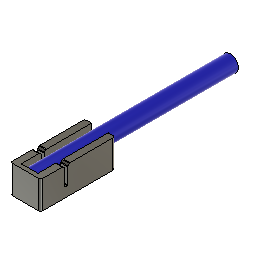
Prusa_MK3_Silicone-Leveling-Jig (Autodesk Fusion 360 design; units mm, degrees)
Autodesk Fusion 360 part; units mm, degrees
sketch "Sketch1" plane through (0, 0, 0) normal (0, 1, 0) x (1, 0, 0)
  circle A0 centre (0, 0) radius 4
  circle A1 centre (0, 0) radius 1.5
  dimension "d1" = 8
  dimension "d2" = 3
  constraint coincident A0.centre A1.centre
  measures "d1" diameter of A0
  measures "d2" diameter of A1
extrude "Extrude1" add sketch "Sketch1" along normal blind 100 makes body 1
sketch "Sketch2" plane through (0, 0, 0) normal (0, 1, 0) x (1, 0, 0)
  circle A0 centre (0, 0) radius 4.15
  line L0 (0, 0) -> (7.5, 0)
  line L1 (7.5, 0) -> (7.5, -7.5)
  line L2 (7.5, -7.5) -> (0, -7.5)
  line L3 (0, -7.5) -> (0, 0)
  line L4 (0, 0) -> (-7.5, 0)
  line L5 (-7.5, 0) -> (-7.5, 7.5)
  line L6 (-7.5, 7.5) -> (0, 7.5)
  line L7 (0, 7.5) -> (0, 0)
  line L8 (-7.5, 7.5) -> (7.5, 7.5)
  line L9 (7.5, 7.5) -> (7.5, -7.5)
  line L10 (7.5, -7.5) -> (-7.5, -7.5)
  line L11 (-7.5, -7.5) -> (-7.5, 7.5)
  dimension "d5" = 8.3
  dimension "d6" = 7.5
  dimension "d7" = 7.5
  dimension "d8" = 7.5
  constraint coincident A0.centre L0.start
  constraint horizontal L0
  constraint vertical L1
  constraint horizontal L2
  constraint vertical L3
  constraint horizontal L4
  constraint vertical L5
  constraint horizontal L6
  constraint vertical L7
  constraint horizontal L8
  constraint vertical L9
  constraint horizontal L10
  constraint vertical L11
  measures "d5" diameter of A0
  measures "d6" distance of A0.centre L0.end
  measures "d7" distance of A0.centre L4.end
  measures "d8" distance of A0.centre L6.end
extrude "Extrude2" add sketch "Sketch2" along normal blind 35 separate body contours A0 L0 L7 L8 L9 | A0 L4 L5 L6 L7 L8 L11 makes body 2
extrude "Extrude3" add 2 faces at (5.2667, 11.6667, 0) (-5.2667, 23.3333, 0) along direction (0, 0, 1) blind 4.5 on bodies 2 bodies 2
sketch "Sketch3" plane through (0, 0, 0) normal (0, -1, 0) x (1, 0, 0)
  arc A0 (-4.15, 0) -> (4.15, 0) centre (0, 0) ccw
  line L0 (-4.15, 0) -> (-4.15, 4.5)
  line L1 (-4.15, 4.5) -> (-7.5, 4.5)
  line L2 (-7.5, 4.5) -> (-7.5, -7.5)
  line L3 (-7.5, -7.5) -> (7.5, -7.5)
  line L4 (7.5, -7.5) -> (7.5, 4.5)
  line L5 (7.5, 4.5) -> (4.15, 4.5)
  line L6 (4.15, 4.5) -> (4.15, 0)
  line L7 (7.5, -7.5) -> (-7.5, -7.5)
  line L8 (-7.5, -7.5) -> (-7.5, 4.5)
  line L9 (-7.5, 4.5) -> (7.5, 4.5)
  line L10 (7.5, 4.5) -> (7.5, -7.5)
  constraint horizontal L7
  constraint vertical L8
  constraint horizontal L9
  constraint vertical L10
  constraint coincident L1.end L2.start
  constraint coincident L3.end L4.start
extrude "Extrude4" add sketch "Sketch3" along normal blind 2 bodies 2
sketch "Sketch4" plane through (0, 0, 4.5) normal (0, 0, 1) x (-1, 0, 0)
  line L0 (4.15, 0) -> (4.15, -35)
  line L1 (4.15, -35) -> (7.5, -35)
  line L2 (7.5, -35) -> (7.5, 2)
  line L3 (7.5, 2) -> (-7.5, 2)
  line L4 (-7.5, 2) -> (-7.5, -35)
  line L5 (-7.5, -35) -> (-4.15, -35)
  line L6 (-4.15, -35) -> (-4.15, 0)
  line L7 (-4.15, 0) -> (4.15, 0)
  line L8 (4.15, 0) -> (4.15, -10)
  line L9 (7.5, -10) -> (-7.5, -10)
  line L10 (-7.5, -10) -> (-7.5, -11.4)
  line L11 (-7.5, -11.4) -> (7.5, -11.4)
  line L12 (7.5, -11.4) -> (7.5, -10)
  dimension "d15" = 10
  dimension "d16" = 15
  dimension "d17" = 1.4
  constraint coincident L0.start L7.end
  constraint perpendicular L7 L8
  constraint horizontal L9
  constraint vertical L10
  constraint horizontal L11
  constraint vertical L12
  constraint coincident L2 L9.start
  measures "d15" distance of L0.start L8.end
  measures "d16" distance of L9.start L9.end
  measures "d17" distance of L9.start L11.end
extrude "Extrude5" cut sketch "Sketch4" against normal blind 9 contours L0 L2 L9 L11 L12 | L0 L6 L9 L11 | L4 L6 L9 L10 L11 bodies 2
extrude "Extrude6" cut 1 faces at (-2.5, 10.9333, -4.5) along direction (0, 0, -1) blind 0.3 on bodies 2 bodies 2
extrude "Extrude7" add 1 faces at (2.5, 10.3333, -7.5) along direction (0, 0, -1) blind 2 on bodies 2 bodies 2
chamfer "Chamfer1" distance 1 angle 45 4 edges at (-5.825, 11.4, 4.5) (-5.825, 10, 4.5) (5.825, 11.4, 4.5) (5.825, 10, 4.5) on bodies 2
fillet "Fillet1" radius 1 4 edges at (7.5, -2, -2.5) (-7.5, -2, -2.5) (7.5, 35, -2.5) (-7.5, 35, -2.5) on bodies 2
fillet "Fillet2" radius 0.5 8 edges at (5.825, 9, 4.5) (5.825, 10, 3.5) (5.825, 11.4, 3.5) (5.825, 12.4, 4.5) (-5.825, 12.4, 4.5) (-5.825, 11.4, 3.5) (-5.825, 10, 3.5) (-5.825, 9, 4.5) on bodies 2
fillet "Fillet3" radius 0.2 2 edges at (0, 11.4, -4.8) (0, 10, -4.8) on bodies 2
fillet "Fillet4" radius 0.1 3 edges at (-4.15, 0, 2.25) (0, 0, -4.15) (4.15, 0, 2.25) on bodies 2
fillet "Fillet5" radius 0.1 3 edges at (-4.15, 35, 2.25) (0, 35, -4.15) (4.15, 35, 2.25) on bodies 2
